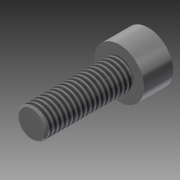
# Autodesk Inventor part: SHCS5x15
Saved by Autodesk Inventor 2015 SP1 (Build 190203100, 203)
## iProperties
Category: Hardware
Created: 2013-12-08
Part Number: SHCS5x15
Material: Stainless Steel
Document SubType Name: Modeling
Designer: Jack
Density: 8.08 g/cm^3
Appearance: Semi-Polished
Vendor: Misumi
Stock Number: CB5-15
Catalog Web Link: http://us.misumi-ec.com/vona2/detail/110300239070/
Author: Jack
Title: SHCS 5x15
Autodesk Inventor part; units mm, degrees
ref_plane "YZ Plane" through (0, 0, 0) normal (1, 0, 0) x (0, 1, 0)
ref_plane "XZ Plane" through (0, 0, 0) normal (0, 1, 0) x (-1, 0, 0)
ref_plane "XY Plane" through (0, 0, 0) normal (0, 0, 1) x (1, 0, 0)
sketch "Sketch1" plane through (0, 0, 0) normal (0, 1, 0) x (-1, 0, 0)
  circle A0 centre (0, 0) radius 2.5
  dimension "d0" = 5
  constraints: 1 centre point, 1 coincident
  measures "d0" diameter of A0
extrude "Extrusion1" add sketch "Sketch1" along normal blind 15
sketch "Sketch2" plane through (0, 15, 0) normal (0, 1, 0) x (1, 0, 0)
  circle A0 centre (0, 0) radius 2.5 projected
  circle A1 centre (0, 0) radius 4.25
  dimension "d3" = 8.5
  constraints: 1 centre point, 1 coincident
  measures "d3" diameter of A1
extrude "Extrusion2" add sketch "Sketch2" along normal blind 5 contours A0 | A1
sketch "Sketch3" plane through (0, 20, 0) normal (0, 1, 0) x (1, 0, 0)
  circle A0 centre (0, 0) radius 4.25 projected
  line L0 (0, 2.3094) -> (2, 1.1547)
  line L1 (2, 1.1547) -> (2, -1.1547)
  line L2 (2, -1.1547) -> (0, -2.3094)
  line L3 (0, -2.3094) -> (-2, -1.1547)
  line L4 (-2, -1.1547) -> (-2, 1.1547)
  line L5 (-2, 1.1547) -> (0, 2.3094)
  dimension "d6" = 2
  constraints: 12 end point, 1 coincident, 1 vertical, 13 other
  measures "d6" distance from line of point (0, 0) L4
extrude "Extrusion3" cut sketch "Sketch3" against normal blind 3.2 contours L0 L1 L2 L3 L4 L5
thread "Thread1" size "M5x0.8" class "6g" standard "ANSI Metric M Profile" full length
chamfer "Chamfer1" distance 0.25 angle 45 1 edges at (2.5, 0, 0)
body "Solid1"
